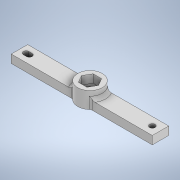
# Autodesk Inventor part: Stützelement
Saved by Autodesk Inventor 2021 (Build 250183000, 183)
## iProperties
Created: 2020-07-18
Part Number: Stützelement
Material: Generisch
Document SubType Name: Modeling
Designer: chris
Density: 1 g/cm^3
Appearance: Vorgabe
Author: chris
Autodesk Inventor part; units mm, degrees
ref_plane "YZ Plane" through (0, 0, 0) normal (1, 0, 0) x (0, 1, 0)
ref_plane "XZ Plane" through (0, 0, 0) normal (0, 1, 0) x (-1, 0, 0)
ref_plane "XY Plane" through (0, 0, 0) normal (0, 0, 1) x (1, 0, 0)
sketch "Skizze1" plane through (0, 0, 0) normal (0, 1, 0) x (-1, 0, 0)
  line L0 (43, -5) -> (-43, -5)
  line L1 (-43, -5) -> (-43, 5)
  line L2 (-43, 5) -> (43, 5)
  line L3 (43, 5) -> (43, -5)
  line L4 (0, -7) -> (0, 7) projected
  line L5 (60.2, 0) -> (-60.2, 0) projected
  point P0 (0, 0)
  dimension "d0" = 10
  dimension "d1" = 86
  constraints: 8 end point, 2 parallel, 1 horizontal, 1 perpendicular, 2 other
  measures "d0" distance of L0.end L1.end
  measures "d1" distance of L1.end L2.end
extrude "Extrusion1" add sketch "Skizze1" along normal blind 5
sketch "Skizze2" plane through (0, 0, 0) normal (0, 1, 0) x (-1, 0, 0)
  circle A0 centre (0, 0) radius 7.5
  dimension "d5" = 15
  constraints: 1 centre point, 1 coincident
  measures "d5" diameter of A0
extrude "Extrusion2" add sketch "Skizze2" along normal blind 10
sketch "Skizze3" plane through (0, 10, 0) normal (0, 1, 0) x (1, 0, 0)
  line L0 (2.5981, 4.5) -> (5.1962, 0)
  line L1 (5.1962, 0) -> (2.5981, -4.5)
  line L2 (2.5981, -4.5) -> (-2.5981, -4.5)
  line L3 (-2.5981, -4.5) -> (-5.1962, 0)
  line L4 (-5.1962, 0) -> (-2.5981, 4.5)
  line L5 (-2.5981, 4.5) -> (2.5981, 4.5)
  point P0 (0, 0)
  point P1 (0, 0)
  dimension "d8" = 9
  constraints: 12 end point, 1 coincident, 1 horizontal, 13 other
  measures "d8" distance between parallel lines of L2 L5
extrude "Extrusion3" cut sketch "Skizze3" against normal blind 5
sketch "Skizze4" plane through (0, 0, 0) normal (0, -1, 0) x (1, 0, 0)
  circle A0 centre (0, 0) radius 2.75
  dimension "d11" = 5.5
  constraints: 1 centre point, 1 coincident
  measures "d11" diameter of A0
extrude "Extrusion4" cut sketch "Skizze4" against normal through all
sketch "Skizze5" plane through (0, 0, 0) normal (0, -1, 0) x (1, 0, 0)
  circle A0 centre (38, 0) radius 1.7
  line L0 (-60.2, 0) -> (60.2, 0) projected
  line L1 (43, 5) -> (43, -5) projected
  line L2 (0, -10.5) -> (0, 10.5) projected
  line L3 (-39, 0) -> (-37, 0) construction
  line L4 (-39, -1.7) -> (-37, -1.7)
  line L5 (-37, 1.7) -> (-39, 1.7)
  arc A1 (-39, 1.7) -> (-39, -1.7) centre (-39, 0) ccw
  arc A2 (-37, -1.7) -> (-37, 1.7) centre (-37, 0) ccw
  line L6 (-43, -5) -> (-43, 5) projected
  point P0 (0, 0)
  point P1 (-38, 0)
  dimension "d14" = 5
  dimension "d15" = 3.4
  dimension "d16" = 5
  dimension "d18" = 3.4
  dimension "d19" = 2
  constraints: 8 end point, 4 point on circle, 4 tangent, 3 centre point, 3 point on line, 1 midpoint, 1 parallel
  measures "d14" distance from line of A0.centre L1
  measures "d15" diameter of A0
  measures "d16" distance from line of point (-38, 0) L6
  measures "d18" distance between parallel lines of L4 L5
  measures "d19" distance of L3.end L3.start
extrude "Extrusion5" cut sketch "Skizze5" against normal through all
fillet "Rundung1" radius 2 7 edges at (7.5, 5, 0) (-7.0063, 5, 2.6762) (-7.0063, 5, -2.6762) (-5.5902, 2.5, 5) (5.5902, 2.5, 5) (5.5902, 2.5, -5) (-5.5902, 2.5, -5)
